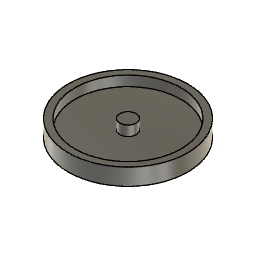
Charger v1 (Autodesk Fusion 360 design; units mm, degrees)
Autodesk Fusion 360 part; units mm, degrees
sketch "Sketch1" plane through (0, 0, 0) normal (0, 0, 1) x (1, 0, 0)
  circle A0 centre (0, 0) radius 7.925
  circle A1 centre (0, 0) radius 8.925
  dimension "d1" = 15.85
  dimension "d4" = 1
  constraint coincident A0.centre A1.centre
  measures "d1" diameter of A0
extrude "Extrude1" add sketch "Sketch1" along normal blind 1 contours A0 | A1
sketch "Sketch2" plane through (0, 0, 1) normal (0, 0, 1) x (-1, 0, 0)
  circle A0 centre (0, 0) radius 8.925
  circle A1 centre (0, 0) radius 7.925
  circle A2 centre (0, 0) radius 1.225
  dimension "d5" = 2.45
  constraint concentric A1 A2
  measures "d5" diameter of A2
extrude "Extrude2" add sketch "Sketch2" along normal blind 1.5
equation "d1 = ( 31.7 / 2 ) * 1 mm"
equation "d5 = ( 4.9 / 2 ) * 1 mm"
